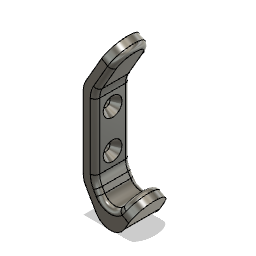
CoatHook_08262021_1633 (Autodesk Fusion 360 design; units mm, degrees)
Autodesk Fusion 360 part; units mm, degrees
sketch "Sketch1" plane through (0, 0, 0) normal (0, 0, 1) x (1, 0, 0)
  line L0 (11.547, 55) -> (0, 35)
  line L1 (0, 35) -> (0, 0)
  line L2 (0, 0) -> (5.4848, -9.5)
  line L3 (17.6092, -9.5) -> (23.094, 0)
  line L4 (15.8771, 52.5) -> (5, 33.6603)
  line L5 (5, 33.6603) -> (5, 1.3397)
  line L6 (5, 1.3397) -> (7.2169, -2.5)
  line L7 (15.8771, -2.5) -> (18.7639, 2.5)
  line L8 (15.8771, 52.5) -> (11.547, 55)
  line L9 (23.094, 0) -> (18.7639, 2.5)
  arc A0 (7.2169, -2.5) -> (15.8771, -2.5) centre (11.547, 0) ccw
  arc A1 (5.4848, -9.5) -> (17.6092, -9.5) centre (11.547, -6) ccw
  point P0 (11.547, -20)
  dimension "d1" = 35
  dimension "d2" = 20
  dimension "d3" = 20
  dimension "d4" = 20
  dimension "d5" = 150
  dimension "d6" = 150
  dimension "d8" = 5
  dimension "d9" = 7
  constraint coincident L1.end L2.start
  constraint vertical L1
  constraint parallel L0 L3
  constraint perpendicular L0 L8
  constraint parallel L0 L4
  constraint parallel L1 L5
  constraint parallel L2 L6
  constraint parallel L3 L7
  constraint tangent L6 A0
  constraint tangent L7 A0
  constraint coincident P0 L2
  constraint coincident P0 L3
  constraint tangent L2 A1
  constraint tangent L3 A1
  measures "d1" distance of L0.end L1.end
  measures "d2" vertical distance of L0.start L0.end
  measures "d3" vertical distance of L1.end P0
  measures "d4" vertical distance of P0 L3.end
  measures "d5" angle of L0 L1
  measures "d6" angle of L1 L2
  measures "d8" radius of A0
  measures "d9" radius of A1
sketch "Sketch2" plane through (0, 0, 0) normal (0, 0, 1) x (1, 0, 0)
sketch "Sketch3" plane through (0, 0, 0) normal (0, 0, 1) x (1, 0, 0)
sketch "Sketch4" plane through (0, 0, 0) normal (0, 0, 1) x (1, 0, 0)
sketch "Sketch5" plane through (0, 0, 0) normal (0, 0, 1) x (1, 0, 0)
sketch "Sketch6" plane through (0, 0, 0) normal (0, 0, 1) x (1, 0, 0)
sketch "Sketch7" plane through (0, 0, 0) normal (0, 0, 1) x (1, 0, 0)
sketch "Sketch8" plane through (0, 0, 0) normal (0, 0, 1) x (1, 0, 0)
extrude "Extrude1" add sketch "Sketch1" along normal blind 15
sketch "Sketch9" plane through (5, 0, 0) normal (1, 0, 0) x (0, 0, -1)
  line L0 (0, 1.3397) -> (0, 33.6603)
  line L1 (0, 33.6603) -> (-15, 33.6603)
  line L2 (-15, 33.6603) -> (-15, 1.3397)
  line L3 (-15, 1.3397) -> (0, 1.3397)
  line L4 (-7.5, 33.6603) -> (-7.5, 1.3397) construction
  line L5 (0, 17.5) -> (-15, 17.5) construction
  circle A0 centre (-7.5, 25.6603) radius 4
  circle A1 centre (-7.5, 9.3397) radius 4
  dimension "d12" = 8
  dimension "d13" = 8
  constraint midpoint L1 L4.start
  constraint midpoint L3 L4.end
  constraint midpoint L0 L5.start
  constraint midpoint L2 L5.end
  constraint coincident L4 A0.centre
  constraint symmetric L5 A0 A1
  measures "d12" diameter of A0
  measures "d13" distance of L4.start A0.centre
extrude "Extrude2" cut sketch "Sketch9" against normal blind 3 draft -35 contours A0 | A1
extrude "Extrude3" cut 2 faces at (2, 25.2296, 7.9641) (2, 8.5998, 6.9769) along direction (-1, 0, 0) through all
fillet "Fillet1" radius 7.5 4 edges at (13.7121, 53.75, 15) (13.7121, 53.75, 0) (20.9289, 1.25, 15) (20.9289, 1.25, 0)
fillet "Fillet2" radius 8 4 edges at (5, 33.6603, 7.5) (5, 1.3397, 7.5) (0, 0, 7.5) (0, 35, 7.5)
fillet "Fillet3" radius 2 16 edges at (5.2726, 33.5872, 15) (9.0995, 40.7607, 15) (15.8771, 52.5, 7.5) (9.0995, 40.7607, 0) (5.2726, 33.5872, 0) (5, 17.5, 0) (5.2726, 1.4128, 0) (6.6443, -1.5083, 0) (10.6702, -4.9225, 0) (15.3815, -3.2072, 0.0512) (18.7639, 2.5, 7.5) (15.3815, -3.2072, 14.9488) (10.6702, -4.9225, 15) (6.6443, -1.5083, 15) (5.2726, 1.4128, 15) (5, 17.5, 15)
equation "d3 = d2"
equation "d4 = d2"
equation "d6 = d5"
